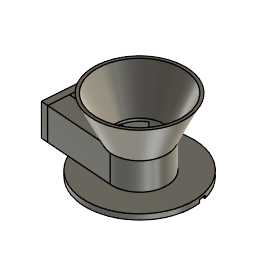
Deckel (Autodesk Fusion 360 design; units mm, degrees)
Autodesk Fusion 360 part; units mm, degrees
cylinder "Grundkörper Zylinder1" add diameter 79 height 4 placed x (1, 0, 0) y (0, 1, 0) z (0, 0, 1) at (0, 0, 0) makes body 1
shell "Schale1" thickness 2 removed faces 1 at (-10.2368, 12.8366, 0) on bodies 1
cylinder "Grundkörper Zylinder2" add diameter 40 height 29.2 placed x (1, 0, 0) y (0, 1, 0) z (0, 0, 1) at (0, 0, 4) separate body makes body 2
move_body "Verschieben17" bodies 2 to x (1, 0, 0) y (0, 1, 0) z (0, 0, 1) at (0, 0, 20)
draft "Verjüngung2" angle 25 neutral plane through (0, 0, 24) pull (0, 0, -1) 1 faces at (19.9006, 1.9914, 33.7333) on bodies 2
extrude "Extrusion4" add 1 faces at (4.7423, -7.1112, 24) along direction (0, 0, -1) blind 20 on bodies 2 bodies 1 2
shell "Schale2" thickness 2 removed faces 2 at (9.3028, 10.3652, 2) at (-3.3884, -3.166, 53.2) on bodies 1
extrude "Extrusion1" cut 1 faces at (30.7934, -2.7573, 2) along direction (0, 0, 1) blind 0.2 on bodies 1 bodies 1
cylinder "Grundkörper Zylinder3" add diameter 67 height 2.2 placed x (0, 1, 0) y (1, 0, 0) z (0, 0, -1) at (0, 0, 2.2) separate body makes body 3
shell "Schale3" thickness 2 outward yes removed faces 2 at (8.7305, 1.9927, 2.2) at (8.7305, 1.9927, 0) on bodies 3
box "Grundkörper Quader1" add length 2.2 width 5 height 8 placed x (0, 0, -1) y (-1, 0, 0) z (0, 1, 0) at (2.5, 0, 2.2) separate body makes body 4
move_body "Verschieben1" bodies 4 to x (1, 0, 0) y (0, 1, 0) z (0, 0, 1) at (0, -40, 0)
move_body "Verschieben5" bodies 4 to x (0.679441, -0.73373, 0) y (0.73373, 0.679441, 0) z (0, 0, 1) at (-1.1803, 0.3346, 0)
combine "Kombinieren5" operation add target body 1 tool bodies 3
combine "Kombinieren1" operation cut target body 1 tool bodies 4 keep tools
move_body "Verschieben3" bodies 4 to x (-0.069756, -0.997564, 0) y (0.997564, -0.069756, 0) z (0, 0, 1) at (-1.3016, -1.5508, 0)
combine "Kombinieren12" operation cut target body 1 tool bodies 4 keep tools
move_body "Verschieben16" bodies 4 to x (-0.461749, -0.887011, 0) y (0.887011, -0.461749, 0) z (0, 0, 1) at (0.4073, -1.0771, 0)
combine "Kombinieren13" operation cut target body 1 tool bodies 4
sketch "Skizze21" plane through (0, 0, 0) normal (0, 0, -1) x (1, 0, 0)
  line L0 (-24.8197, -25.3817) -> (-23.5602, -23.8152)
  arc A0 (-26.8521, 20.0304) -> (-23.5602, -23.8152) centre (0, 0) ccw
  line L1 (-26.8521, 20.0304) -> (-28.3273, 21.3965)
  arc A1 (-28.3273, 21.3965) -> (-24.8197, -25.3817) centre (0, 0) ccw
  line L2 (-23.5602, -23.8152) -> (-26.8521, 20.0304) construction
  line L3 (-26.3289, 13.0655, 6.75) -> (-24.0834, -16.8503, 6.75)
  line L4 (-24.0834, -16.8503, 6.75) -> (-24.0834, -16.8503, -6.75)
  line L5 (-24.0834, -16.8503, -6.75) -> (-26.3289, 13.0655, -6.75)
  line L6 (-26.3289, 13.0655, -6.75) -> (-26.3289, 13.0655, 6.75)
  line L7 (-26.3289, 13.0655, 6.75) -> (-24.0834, -16.8503, -6.75) construction
  line L8 (-24.0834, -16.8503, 6.75) -> (-26.3289, 13.0655, -6.75) construction
  point P0 (-25.2061, -1.8924)
  dimension "d45" = 30
  dimension "d46" = 13.5
  constraint coincident L0.end A0.end
  constraint coincident A0.start L1.start
  constraint midpoint L2 P0
extrude "Extrusion5" add sketch "Skizze21" against normal blind 50 separate body contours L3 L4 L5 L6 in plane through (-25.2062, 1.8921, 0) normal (0.997195, -0.074853, 0) makes body 5
move_body "Verschieben18" bodies 5 to x (1, 0, 0) y (0, 1, 0) z (0, 0, 1) at (24.9569, -1.8737, 15.75)
combine "Kombinieren14" operation cut target body 1 tool bodies 5 keep tools
shell "Schale4" thickness 5 outward yes removed faces 2 at (0.125, 5.0047, 13.5) at (-49.7347, 8.7473, 13.5) on bodies 5
combine "Kombinieren15" operation cut target body 5 tool bodies 1 keep tools makes body 6 at (-40.0726, 2.5123, 4)
delete_body "Körper entfernen3" bodies 5
sketch "Skizze24" plane through (0, 0, 27.5) normal (0, 0, 1) x (-1, 0, 0)
  line L0 (6.7228, -20.5609) -> (48.6119, -23.7052)
  line L1 (48.6119, -23.7052) -> (51.606, 16.1826)
  line L2 (51.606, 16.1826) -> (9.7169, 19.3269)
  line L3 (50.1089, -3.7613) -> (50.4832, 1.2246) construction
  line L4 (50.4832, 1.2246) -> (40.5113, 1.9732)
  line L5 (40.5113, 1.9732) -> (39.7627, -7.9988)
  line L6 (39.7627, -7.9988) -> (49.7347, -8.7473)
  arc A0 (6.7228, -20.5609) -> (9.7169, 19.3269) centre (0, 0) ccw
  dimension "d47" = 5
  dimension "d48" = 10
  dimension "d49" = 10
  constraint midpoint L1 L3.start
  constraint parallel L1 L3
  constraint perpendicular L3 L4
  constraint perpendicular L4 L5
  constraint coincident L1 L6.end
  constraint perpendicular L1 L6
  measures "d47" distance of L3.start L3.end
  measures "d48" distance of L3.end L4.end
  measures "d49" distance of L4.end L5.end
extrude "Extrusion8" cut sketch "Skizze24" against normal blind 5 contours L1 L4 L5 L6 bodies 6
sketch "Skizze26" plane through (-50.1089, 3.7613, 0) normal (-0.997195, 0.074853, 0) x (-0.074853, -0.997195, 0)
  line L0 (5, 27.5) -> (5, 22.5)
  line L1 (5, 22.5) -> (15, 22.5)
  line L2 (15, 22.5) -> (15, 9)
  line L3 (15, 9) -> (-15, 9)
  line L4 (-15, 9) -> (-15, 22.5)
  line L5 (-15, 22.5) -> (-5, 22.5)
  line L6 (-5, 22.5) -> (-5, 27.5)
  line L7 (-5, 27.5) -> (-20, 27.5)
  line L8 (-20, 27.5) -> (-20, 4)
  line L9 (-20, 4) -> (20, 4)
  line L10 (20, 4) -> (20, 27.5)
  line L11 (20, 27.5) -> (5, 27.5)
  line L12 (-5, 27.5) -> (5, 27.5)
  line L13 (20, 27.5) -> (18.75, 27.5) construction
  line L14 (18.75, 27.5) -> (18.75, 26.25) construction
  line L15 (18.75, 26.25) -> (20, 26.25) construction
  line L16 (20, 26.25) -> (20, 27.5) construction
  line L17 (-20, 27.5) -> (-18.75, 27.5) construction
  line L18 (-18.75, 27.5) -> (-18.75, 26.25) construction
  line L19 (-18.75, 26.25) -> (-20, 26.25) construction
  line L20 (-20, 26.25) -> (-20, 27.5) construction
  line L21 (20, 4) -> (18.75, 4) construction
  line L22 (18.75, 4) -> (18.75, 5.25) construction
  line L23 (18.75, 5.25) -> (20, 5.25) construction
  line L24 (20, 5.25) -> (20, 4) construction
  line L25 (-20, 4) -> (-18.75, 4) construction
  line L26 (-18.75, 4) -> (-18.75, 5.25) construction
  line L27 (-18.75, 5.25) -> (-20, 5.25) construction
  line L28 (-20, 5.25) -> (-20, 4) construction
  line L29 (5, 27.5) -> (6.25, 27.5) construction
  line L30 (6.25, 27.5) -> (6.25, 26.25) construction
  line L31 (6.25, 26.25) -> (5, 26.25) construction
  line L32 (5, 26.25) -> (5, 27.5) construction
  line L33 (-5, 27.5) -> (-6.25, 27.5) construction
  line L34 (-6.25, 27.5) -> (-6.25, 26.25) construction
  line L35 (-6.25, 26.25) -> (-5, 26.25) construction
  line L36 (-5, 26.25) -> (-5, 27.5) construction
  line L37 (18.75, 26.25) -> (6.25, 26.25)
  line L38 (6.25, 26.25) -> (6.25, 23.75)
  line L39 (6.25, 23.75) -> (18.75, 23.75)
  line L40 (18.75, 23.75) -> (18.75, 26.25)
  line L41 (-18.75, 26.25) -> (-6.25, 26.25)
  line L42 (-6.25, 26.25) -> (-6.25, 23.75)
  line L43 (-6.25, 23.75) -> (-18.75, 23.75)
  line L44 (-18.75, 23.75) -> (-18.75, 26.25)
  line L45 (18.75, 5.25) -> (-18.75, 5.25)
  line L46 (-18.75, 5.25) -> (-18.75, 7.75)
  line L47 (-18.75, 7.75) -> (18.75, 7.75)
  line L48 (18.75, 7.75) -> (18.75, 5.25)
  line L49 (18.75, 23.75) -> (16.25, 23.75)
  line L50 (16.25, 23.75) -> (16.25, 7.75)
  line L51 (16.25, 7.75) -> (18.75, 7.75)
  line L52 (18.75, 7.75) -> (18.75, 23.75)
  line L53 (-18.75, 23.75) -> (-16.25, 23.75)
  line L54 (-16.25, 23.75) -> (-16.25, 7.75)
  line L55 (-16.25, 7.75) -> (-18.75, 7.75)
  line L56 (-18.75, 7.75) -> (-18.75, 23.75)
  dimension "d54" = 1.25
  dimension "d55" = 1.25
  dimension "d56" = 1.25
  dimension "d57" = 1.25
  dimension "d58" = 1.25
  dimension "d59" = 1.25
  dimension "d60" = 1.25
  dimension "d61" = 1.25
  dimension "d68" = 1.25
  dimension "d69" = 1.25
  dimension "d70" = 1.25
  dimension "d71" = 1.25
  dimension "d72" = 2.5
  dimension "d73" = 2.5
  dimension "d74" = 2.5
  dimension "d75" = 2.5
  dimension "d76" = 2.5
  constraint coincident L6.end L7.start
  constraint coincident L11 L0.start
  constraint horizontal L13
  constraint vertical L14
  constraint horizontal L15
  constraint vertical L16
  constraint coincident L10.end L11.start
  constraint horizontal L17
  constraint vertical L18
  constraint horizontal L19
  constraint vertical L20
  constraint coincident L7.end L8.start
  constraint horizontal L21
  constraint vertical L22
  constraint horizontal L23
  constraint vertical L24
  constraint coincident L9.end L10.start
  constraint horizontal L25
  constraint vertical L26
  constraint horizontal L27
  constraint vertical L28
  constraint coincident L8.end L9.start
  constraint horizontal L29
  constraint vertical L30
  constraint horizontal L31
  constraint vertical L32
  constraint coincident L0.start L11.end
  constraint horizontal L33
  constraint vertical L34
  constraint horizontal L35
  constraint vertical L36
  constraint horizontal L37
  constraint vertical L38
  constraint horizontal L39
  constraint vertical L40
  constraint horizontal L41
  constraint vertical L42
  constraint horizontal L43
  constraint vertical L44
  constraint horizontal L45
  constraint vertical L46
  constraint horizontal L47
  constraint vertical L48
  constraint horizontal L49
  constraint vertical L50
  constraint horizontal L51
  constraint vertical L52
  constraint coincident L47 L50.end
  constraint horizontal L53
  constraint vertical L54
  constraint horizontal L55
  constraint vertical L56
  measures "d54" distance of L10.end L13.end
  measures "d55" distance of L10.end L15.end
  measures "d56" distance of L7.end L17.end
  measures "d57" distance of L7.end L19.end
  measures "d58" distance of L9.end L21.end
  measures "d59" distance of L9.end L23.end
  measures "d60" distance of L8.end L25.end
  measures "d61" distance of L8.end L27.end
  measures "d68" distance of L0.start L29.end
  measures "d69" distance of L0.start L31.end
  measures "d70" distance of L6.end L33.end
  measures "d71" distance of L6.end L35.end
  measures "d72" distance of L14.end L39.end
  measures "d73" distance of L18.end L43.end
  measures "d74" distance of L22.end L47.end
  measures "d75" distance of L39.end L49.end
  measures "d76" distance of L43.end L53.end
combine "Kombinieren17" operation add target body 1 tool bodies 6
extrude "Extrusion9" add sketch "Skizze26" along normal blind 5 separate body contours L0 L1 L2 L3 L4 L5 L6 L7 L8 L9 L10 L11 | L0 L1 L2 L3 L4 L5 L6 L12 | L37 L38 L39 L40 L49 | L39 L47 L49 L50 L51 L52 | L45 L46 L47 L48 L51 L55 | L43 L47 L53 L54 L55 L56 | L41 L42 L43 L44 L53 makes body 7
extrude "Extrusion10" add sketch "Skizze26" against normal blind 5 contours L37 L38 L39 L40 L49 | L39 L47 L49 L50 L51 L52 | L45 L46 L47 L48 L51 L55 | L43 L47 L53 L54 L55 L56 | L41 L42 L43 L44 L53 bodies 7
combine "Kombinieren18" operation cut target body 1 tool bodies 7 keep tools
move_face "Flächen versetzen1" offset -0.125 12 faces at (-49.5386, -10.9058, 26.25) (-49.8504, -15.0608, 12.25) (-47.9791, 9.869, 25.4167) (-48.9148, -2.5959, 25.4167) (-47.3554, 18.179, 26.25) (-45.3815, 22.2092, 12.25) (-46.3171, 9.7443, 5.25) (-48.0415, 9.038, 7.75) (-49.6633, -12.5678, 18.4167) (-47.2306, 19.841, 18.4167) (-47.7296, 13.193, 23.75) (-49.1643, -5.9199, 23.75) on bodies 7
extrude "Extrusion11" cut 1 faces at (-44.7144, 8.8301, 6.125) along direction (-0.997195, 0.074853, 0) blind 0.1 on bodies 7 bodies 7
named bodies: "Oberteil", "Lichtschranken_Kappe"
